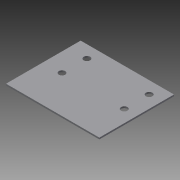
# Autodesk Inventor part: slider
Saved by Autodesk Inventor 2014 SP1 (Build 180222100, 222)
## iProperties
Created: 2014-10-09
Part Number: slider
Material: Generic
Document SubType Name: Modeling
Designer: Rachel
Density: 1 g/cm^3
Appearance: Default
Author: Rachel
Autodesk Inventor part; units mm, degrees
ref_plane "YZ Plane" through (0, 0, 0) normal (1, 0, 0) x (0, 1, 0)
ref_plane "XZ Plane" through (0, 0, 0) normal (0, 1, 0) x (-1, 0, 0)
ref_plane "XY Plane" through (0, 0, 0) normal (0, 0, 1) x (1, 0, 0)
sketch "Sketch1" plane through (0, 0, 0) normal (0, 1, 0) x (-1, 0, 0)
  line L0 (0, 0) -> (95.25, 0)
  line L1 (95.25, 0) -> (95.25, 76.2)
  line L2 (95.25, 76.2) -> (0, 76.2)
  line L3 (0, 76.2) -> (0, 0)
  point P0 (76.2, 12.7)
  point P1 (12.7, 13.1017)
  point P2 (76.2, 38.1)
  point P3 (12.7, 38.1)
  dimension "d0" = 95.25
  dimension "d1" = 76.2
  dimension "d14" = 12.7
  dimension "d15" = 19.05
  dimension "d16" = 63.5
  dimension "d29" = 19.05
  dimension "d30" = 38.1
  dimension "d31" = 63.5
  constraints: 8 end point, 2 parallel, 1 horizontal, 1 perpendicular
  measures "d0" distance of L2.end L1.end
  measures "d1" distance between parallel lines of L0 L2
  measures "d14" distance from line of L0 point (76.2, 12.7)
  measures "d15" distance from line of L1 point (76.2, 12.7)
  measures "d16" horizontal distance of point (76.2, 12.7) point (12.7, 13.102)
  measures "d29" distance from line of L1 point (76.2, 38.1)
  measures "d30" distance from line of L2 point (76.2, 38.1)
  measures "d31" distance of point (76.2, 38.1) point (12.7, 38.1)
extrude "Extrusion2" add sketch "Sketch1" along normal blind 1.5875
sketch "Sketch3" plane through (0, 1.5875, 0) normal (0, 1, 0) x (1, 0, 0)
  line L0 (0, 0) -> (-95.25, 0) projected
  line L1 (-95.25, 0) -> (-95.25, -76.2) projected
  point P0 (-76.2, -12.7)
  point P1 (-12.7, -12.7)
  point P2 (-76.2, -38.1)
  point P3 (-12.7, -38.1)
  dimension "d19" = 19.05
  dimension "d20" = 12.7
  dimension "d21" = 63.5
  dimension "d32" = 25.4
  dimension "d33" = 63.5
  dimension "d34" = 19.05
  measures "d19" distance from line of L1 point (-76.2, -12.7)
  measures "d20" distance from line of L0 point (-76.2, -12.7)
  measures "d21" distance of point (-12.7, -12.7) point (-76.2, -12.7)
  measures "d32" distance of point (-76.2, -12.7) point (-76.2, -38.1)
  measures "d33" distance of point (-12.7, -38.1) point (-76.2, -38.1)
  measures "d34" distance from line of L1 point (-76.2, -38.1)
hole "Hole3" at (-76.2, 1.5875, 12.7) at (-12.7, 1.5875, 12.7) at (-76.2, 1.5875, 38.1) at (-12.7, 1.5875, 38.1) direction (0, -1, 0) diameter 6.477 end through all
body "Solid2"
